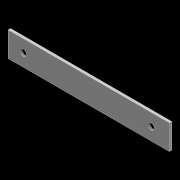
# Autodesk Inventor part: lastflat bar
Saved by Autodesk Inventor 2016 (Build 200138000, 138)
## iProperties
Created: 2019-02-12
Part Number: lastflat bar
Material: Generic
Document SubType Name: Modeling
Designer: Calb3e
Density: 1 g/cm^3
Appearance: Default
Author: Calb3e
Autodesk Inventor part; units mm, degrees
ref_plane "YZ Plane" through (0, 0, 0) normal (1, 0, 0) x (0, 1, 0)
ref_plane "XZ Plane" through (0, 0, 0) normal (0, 1, 0) x (-1, 0, 0)
ref_plane "XY Plane" through (0, 0, 0) normal (0, 0, 1) x (1, 0, 0)
sketch "Sketch1" plane through (0, 0, 0) normal (0, 1, 0) x (-1, 0, 0)
  line L0 (0, 0) -> (-130, 0)
  line L1 (-130, 0) -> (-130, 20)
  line L2 (-130, 20) -> (0, 20)
  line L3 (0, 20) -> (0, 0)
  dimension "d0" = 130
  dimension "d1" = 20
  constraints: 8 end point, 2 parallel, 1 horizontal, 1 perpendicular
  measures "d0" distance of L1.end L2.end
  measures "d1" distance of L2.end L0.start
extrude "Extrusion1" add sketch "Sketch1" along normal blind 2
hole "Hole1" at (12, 2, 10) direction (0, -1, 0) diameter 5.5 end through all
pattern_linear "Rectangular Pattern1" count 2 spacing 103.172 along (1, 0, 0) of "Hole1"
body "Solid1"
